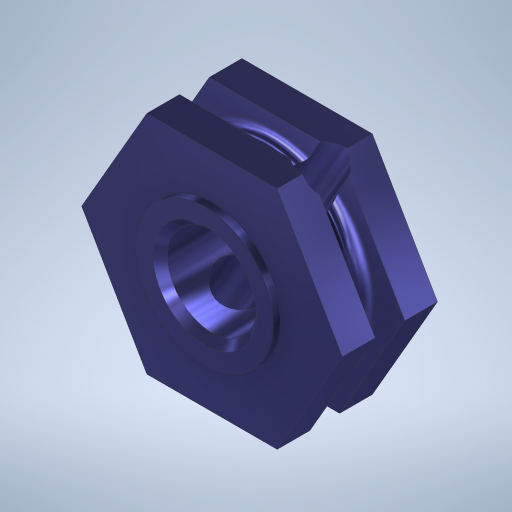
# Autodesk Inventor part: Hex Drive
Saved by Autodesk Inventor 2023.1 (Build 271208000, 208)
## iProperties
Created: 2019-11-19
Part Number: Hex Drive
Material: Generic
Document SubType Name: Modeling
Designer: Jopa
Density: 1 g/cm^3
Appearance: Default
Author: Jopa
Autodesk Inventor part; units mm, degrees
ref_plane "YZ Plane" through (0, 0, 0) normal (1, 0, 0) x (0, 1, 0)
sketch "Sketch1" plane through (0, 0, 0) normal (0, 0, 1) x (1, 0, 0)
  circle A0 centre (0, 0) radius 6.0325 construction
  line L0 (3.4829, 6.0325) -> (6.9657, 0)
  line L1 (6.9657, 0) -> (3.4829, -6.0325)
  line L2 (3.4829, -6.0325) -> (-3.4829, -6.0325)
  line L3 (-3.4829, -6.0325) -> (-6.9657, 0)
  line L4 (-6.9657, 0) -> (-3.4829, 6.0325)
  line L5 (-3.4829, 6.0325) -> (3.4829, 6.0325)
  point P0 (0, 6.0325)
  dimension "d0" = 12.065
  constraints: 12 end point, 2 coincident, 1 horizontal, 1 midpoint, 1 vertical alignment, 15 other
extrude "Extrusion1" add sketch "Sketch1" along normal mid plane 5.08
sketch "Sketch2" plane through (0, 0, 2.54) normal (0, 0, 1) x (1, 0, 0)
  circle A0 centre (0, 0) radius 2.3813
  circle A1 centre (0, 0) radius 3.6513
  dimension "d3" = 4.7625
  dimension "d4" = 1.27
  constraints: 2 centre point, 1 coincident
  measures "d3" diameter of A0
  measures "d4" radial gap between concentric circles of A1 A0
extrude "Extrusion2" add sketch "Sketch2" along normal blind 0.381
extrude "Extrusion3" cut sketch "Sketch2" against normal through all contours A0
chamfer "Chamfer1" distance 0.381 angle 45 1 edges at (-2.3813, 0, 2.921)
ref_plane "Work Plane1" through (3.4829, 6.0325, 0) normal (0.5, 0.866, 0) x (0, 0, 1)
sketch "Sketch3" plane through (3.4829, 6.0325, 0) normal (0.5, 0.866, 0) x (0, 0, 1)
  circle A0 centre (0, 0) radius 1.1913
  dimension "d13" = 2.3825
  constraints: 1 centre point, 1 coincident
  measures "d13" diameter of A0
extrude "Extrusion4" cut sketch "Sketch3" against normal through all
ref_plane "Work Plane2" through (3.4829, 6.0325, 0) normal (0.866, -0.5, 0) x (0, 0, 1)
sketch "Sketch4" plane through (3.4829, 6.0325, 0) normal (0.866, -0.5, 0) x (0, 0, 1)
  line L0 (-1.1913, 4.5845) -> (-1.1913, 0) construction
  line L1 (-1.1913, 0) -> (-2.54, 0) construction
  line L2 (-2.54, 0) -> (-2.54, 4.5845) construction
  line L3 (-2.54, 4.5845) -> (-1.1913, 4.5845) construction
  line L4 (-1.1913, 13.9315) -> (-1.1913, 9.347) construction
  line L5 (-1.1913, 9.347) -> (-2.54, 9.347) construction
  line L6 (-2.54, 9.347) -> (-2.54, 13.9315) construction
  line L7 (-2.54, 13.9315) -> (-1.1913, 13.9315) construction
  line L8 (2.921, 9.728) -> (2.54, 9.347) construction
  line L9 (2.54, 9.347) -> (1.1913, 9.347) construction
  line L10 (1.1913, 9.347) -> (1.1913, 13.9315) construction
  line L11 (1.1913, 13.9315) -> (2.54, 13.9315) construction
  line L12 (2.54, 13.9315) -> (2.54, 10.617) construction
  line L13 (2.54, 10.617) -> (2.921, 10.617) construction
  line L14 (2.921, 10.617) -> (2.921, 9.728) construction
  line L15 (2.54, 4.5845) -> (2.921, 4.2035) construction
  line L16 (2.921, 4.2035) -> (2.921, 3.3145) construction
  line L17 (2.921, 3.3145) -> (2.54, 3.3145) construction
  line L18 (2.54, 3.3145) -> (2.54, 0) construction
  line L19 (2.54, 0) -> (1.1913, 0) construction
  line L20 (1.1913, 0) -> (1.1913, 4.5845) construction
  line L21 (1.1913, 4.5845) -> (2.54, 4.5845) construction
  line L22 (-0.7937, 0) -> (-0.7937, 1.5875)
  arc A0 (0.7938, 1.5875) -> (-0.7937, 1.5875) centre (0, 1.5875) ccw
  line L23 (0.7938, 1.5875) -> (0.7938, 0)
  line L24 (0.7938, 0) -> (-0.7937, 0)
  line L25 (-3.6322, 6.9657) -> (4.0132, 6.9657) projected
  point P0 (0, 6.9657)
  dimension "d16" = 1.5875
  dimension "d17" = 1.5875
  constraints: 6 end point, 2 point on circle, 2 tangent, 1 centre point, 1 collinear, 1 parallel, 1 perpendicular, 1 vertical, 1 vertical alignment
  measures "d16" diameter of A0
  measures "d17" distance from line of L24 A0.centre
revolve "Revolution1" cut sketch "Sketch4" angle 360 about axis through (0, 0, -10) along (0, 0, 1)
equation "\"d17\" = d16"
body "Solid1"
